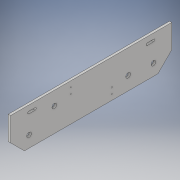
# Autodesk Inventor part: DriveTrain3.0
Saved by Autodesk Inventor 2017 (Build 210142000, 142)
## iProperties
Created: 2017-07-22
Part Number: DriveTrain3.0
Material: Generic
Document SubType Name: Modeling
Designer: User
Density: 1 g/cm^3
Appearance: Default
Author: User
Autodesk Inventor part; units mm, degrees
ref_plane "YZ Plane" through (0, 0, 0) normal (1, 0, 0) x (0, 1, 0)
ref_plane "XZ Plane" through (0, 0, 0) normal (0, 1, 0) x (-1, 0, 0)
ref_plane "XY Plane" through (0, 0, 0) normal (0, 0, 1) x (1, 0, 0)
sketch "Sketch1" plane through (0, 0, 0) normal (1, 0, 0) x (0, 1, 0)
  line L0 (0, 0) -> (103.378, 0)
  line L1 (103.378, 0) -> (103.378, -444.5)
  line L2 (103.378, -444.5) -> (0, -444.5)
  line L3 (0, -444.5) -> (0, 0)
  circle A0 centre (31.75, -50.8) radius 6.3627
  circle A1 centre (31.75, -393.7) radius 6.3627
  circle A2 centre (88.0618, -165.5318) radius 1.5875
  circle A3 centre (72.0598, -165.5318) radius 1.5875
  circle A4 centre (15.3162, -278.9682) radius 1.5875
  circle A5 centre (31.3182, -278.9682) radius 1.5875
  dimension "d0" = 103.378
  dimension "d1" = 444.5
  dimension "d2" = 12.7254
  dimension "d3" = 31.75
  dimension "d4" = 50.8
  dimension "d5" = 50.8
  dimension "d22" = 165.5318
  dimension "d23" = 3.175
  dimension "d24" = 15.3162
  dimension "d25" = 3.175
  dimension "d26" = 16.002
  dimension "d27" = 165.5318
  dimension "d28" = 3.175
  dimension "d29" = 15.3162
  dimension "d30" = 165.5318
  dimension "d31" = 3.175
  dimension "d32" = 16.002
  dimension "d33" = 165.5318
  constraints: 8 end point, 6 centre point, 2 parallel, 1 horizontal, 1 perpendicular
  measures "d0" distance of L1.end L2.end
  measures "d1" distance of L0.end L1.end
  measures "d2" diameter of A0
  measures "d3" distance from line of L3 A0.centre
  measures "d4" distance from line of L0 A0.centre
  measures "d5" distance from line of L2 A1.centre
  measures "d22" distance from line of L0 A2.centre
  measures "d23" diameter of A2
  measures "d24" distance from line of L1 A2.centre
  measures "d25" diameter of A3
  measures "d26" distance of A2.centre A3.centre
  measures "d27" distance from line of L0 A3.centre
  measures "d28" diameter of A4
  measures "d29" distance from line of L3 A4.centre
  measures "d30" distance from line of L2 A4.centre
  measures "d31" diameter of A5
  measures "d32" distance of A5.centre A4.centre
  measures "d33" distance from line of L2 A5.centre
extrude "Extrusion1" add sketch "Sketch1" along normal blind 6.35 contours L0 L1 L2 L3 | A2 | A3 | A4 | A5
chamfer "Chamfer1" distance 38.1 angle 45 1 edges at (3.175, 0, 0)
chamfer "Chamfer2" distance 38.1 angle 45 1 edges at (3.175, 0, -444.5)
sketch "Sketch2" plane through (6.35, 0, 0) normal (1, 0, 0) x (0, 0, -1)
  line L0 (444.5, 38.1) -> (406.4, 0) projected
  line L1 (444.5, 38.1) -> (444.5, 103.378) projected
  line L2 (444.5, 103.378) -> (0, 103.378) projected
  line L3 (0, 103.378) -> (0, 38.1) projected
  line L4 (38.1, 0) -> (0, 38.1) projected
  line L5 (38.1, 0) -> (406.4, 0) projected
  circle A0 centre (393.7, 31.75) radius 6.3627 projected
  circle A1 centre (50.8, 31.75) radius 6.3627 projected
  circle A2 centre (120.4214, 66.0654) radius 6.3627
  circle A3 centre (324.0786, 37.3126) radius 6.3627
  point P0 (0, 0)
  dimension "d14" = 12.7254
  dimension "d15" = 120.4214
  dimension "d16" = 37.3126
  dimension "d17" = 12.7254
  dimension "d18" = 37.3126
  dimension "d19" = 120.4214
  constraints: 2 centre point
  measures "d14" diameter of A2
  measures "d15" distance from line of L3 A2.centre
  measures "d16" distance from line of L2 A2.centre
  measures "d17" diameter of A3
  measures "d18" distance from line of L5 A3.centre
  measures "d19" distance from line of L1 A3.centre
extrude "Extrusion2" cut sketch "Sketch2" against normal blind 25.4 contours A2 | A3
sketch "Sketch3" plane through (6.35, 0, 0) normal (1, 0, 0) x (0, 0, -1)
  circle A0 centre (120.4214, 66.0654) radius 6.3627 projected
  circle A1 centre (324.0786, 37.3126) radius 6.3627 projected
  line L0 (444.5, 38.1) -> (406.4, 0) projected
  line L1 (444.5, 38.1) -> (444.5, 103.378) projected
  line L2 (444.5, 103.378) -> (0, 103.378) projected
  line L3 (0, 103.378) -> (0, 38.1) projected
  line L4 (38.1, 0) -> (0, 38.1) projected
  line L5 (38.1, 0) -> (406.4, 0) projected
  circle A2 centre (393.7, 31.75) radius 6.3627 projected
  circle A3 centre (50.8, 31.75) radius 6.3627 projected
  circle A4 centre (165.5318, 88.0618) radius 1.5875
  circle A5 centre (165.5318, 72.0598) radius 1.5875
  circle A6 centre (278.9682, 15.3162) radius 1.5875
  circle A7 centre (278.9682, 31.3182) radius 1.5875
  point P0 (0, 0)
  dimension "d34" = 3.175
  dimension "d35" = 165.5318
  dimension "d36" = 15.3162
  dimension "d37" = 3.175
  dimension "d38" = 16.002
  dimension "d39" = 3.175
  dimension "d40" = 3.175
  dimension "d41" = 15.3162
  dimension "d42" = 16.002
  dimension "d43" = 165.5318
  constraints: 4 centre point
  measures "d34" diameter of A4
  measures "d35" distance from line of L3 A4.centre
  measures "d36" distance from line of L2 A4.centre
  measures "d37" diameter of A5
  measures "d38" distance of A4.centre A5.centre
  measures "d39" diameter of A6
  measures "d40" diameter of A7
  measures "d41" distance from line of L5 A6.centre
  measures "d42" distance of A7.centre A6.centre
  measures "d43" distance from line of L1 A6.centre
extrude "Extrusion3" cut sketch "Sketch3" against normal blind 25.4 contours A4 | A5 | A6 | A7
sketch "Sketch4" plane through (6.35, 0, 0) normal (1, 0, 0) x (0, 0, -1)
  circle A0 centre (278.9682, 15.3162) radius 1.5875 projected
  circle A1 centre (165.5318, 88.0618) radius 1.5875 projected
  circle A2 centre (165.5318, 72.0598) radius 1.5875 projected
  circle A3 centre (278.9682, 31.3182) radius 1.5875 projected
  circle A4 centre (120.4214, 66.0654) radius 6.3627 projected
  circle A5 centre (324.0786, 37.3126) radius 6.3627 projected
  line L0 (444.5, 38.1) -> (406.4, 0) projected
  line L1 (444.5, 38.1) -> (444.5, 103.378) projected
  line L2 (444.5, 103.378) -> (0, 103.378) projected
  line L3 (0, 103.378) -> (0, 38.1) projected
  line L4 (38.1, 0) -> (0, 38.1) projected
  line L5 (38.1, 0) -> (406.4, 0) projected
  circle A6 centre (393.7, 31.75) radius 6.3627 projected
  circle A7 centre (50.8, 31.75) radius 6.3627 projected
  arc A8 (50.165, 88.773) -> (50.165, 82.423) centre (50.165, 85.598) ccw
  arc A9 (67.31, 82.423) -> (67.31, 88.773) centre (67.31, 85.598) ccw
  line L6 (50.165, 82.423) -> (67.31, 82.423)
  line L7 (67.31, 88.773) -> (50.165, 88.773)
  arc A10 (394.335, 82.423) -> (394.335, 88.773) centre (394.335, 85.598) ccw
  arc A11 (377.19, 88.773) -> (377.19, 82.423) centre (377.19, 85.598) ccw
  line L8 (377.19, 82.423) -> (394.335, 82.423)
  line L9 (394.335, 88.773) -> (377.19, 88.773)
  point P0 (0, 0)
  dimension "d46" = 6.35
  dimension "d47" = 50.165
  dimension "d48" = 17.78
  dimension "d49" = 6.35
  dimension "d50" = 17.145
  dimension "d51" = 6.35
  dimension "d52" = 50.165
  dimension "d53" = 17.78
  dimension "d54" = 6.35
  dimension "d56" = 17.145
  constraints: 8 end point, 8 point on circle, 4 centre point, 2 horizontal, 2 parallel
  measures "d46" diameter of A8
  measures "d47" distance from line of L3 A8.centre
  measures "d48" distance from line of L2 A8.centre
  measures "d49" diameter of A9
  measures "d50" distance of A9.centre A8.centre
  measures "d51" diameter of A10
  measures "d52" distance from line of L1 A10.centre
  measures "d53" distance from line of L2 A10.centre
  measures "d54" diameter of A11
  measures "d56" distance of L8.start L8.end
extrude "Extrusion4" cut sketch "Sketch4" against normal blind 25.4 contours L7 A9 L6 A8 | L8 A11 L9 A10
body "Solid1"
